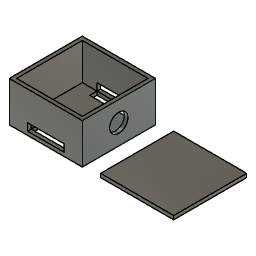
Caja Prototipo 1 v1 (Autodesk Fusion 360 design; units mm, degrees)
Autodesk Fusion 360 part; units mm, degrees
sketch "Boceto1" plane through (0, 0, 0) normal (0, 0, 1) x (1, 0, 0)
  line L0 (100, 100) -> (-100, 100)
  line L1 (-100, 100) -> (-100, -100)
  line L2 (-100, -100) -> (100, -100)
  line L3 (100, -100) -> (100, 100)
  line L4 (100, 100) -> (-100, -100) construction
  line L5 (-100, 100) -> (100, -100) construction
  dimension "L_base" = 200
  constraint horizontal L0
  constraint perpendicular L0 L1
  constraint parallel L0 L2
  constraint parallel L1 L3
  constraint coincident L4 origin
  constraint coincident L5 origin
  constraint equal L0 L1
  measures "L_base" distance of L0.end L1.end
extrude "Extruir1" add sketch "Boceto1" along normal blind 10 makes body 1
sketch "Boceto2" plane through (0, 0, 10) normal (0, 0, 1) x (-1, 0, 0)
  line L0 (-100, 100) -> (-100, -100)
  line L1 (-100, -100) -> (100, -100)
  line L2 (100, -100) -> (100, 100)
  line L3 (100, 100) -> (-100, 100)
  line L4 (100, -100) -> (90, -100)
  line L5 (90, -100) -> (90, 100)
  line L6 (90, 100) -> (100, 100)
  line L7 (100, 100) -> (100, -100)
  line L8 (90, -90) -> (-100, -90)
  line L9 (-100, -90) -> (-100, -100)
  line L10 (-100, -100) -> (90, -100)
  line L11 (90, -100) -> (90, -90)
  line L12 (-90, -90) -> (-100, -90)
  line L13 (-100, -90) -> (-100, 100)
  line L14 (-100, 100) -> (-90, 100)
  line L15 (-90, 100) -> (-90, -90)
  line L16 (-90, 100) -> (90, 100)
  line L17 (90, 100) -> (90, 90)
  line L18 (90, 90) -> (-90, 90)
  line L19 (-90, 90) -> (-90, 100)
  dimension "d4" = 10
  dimension "d5" = 10
  dimension "d6" = 10
  dimension "d7" = 10
  constraint horizontal L4
  constraint vertical L5
  constraint horizontal L6
  constraint vertical L7
  constraint coincident L3 L5.end
  constraint coincident L1.end L2.start
  constraint horizontal L8
  constraint vertical L9
  constraint horizontal L10
  constraint vertical L11
  constraint coincident L0.end L1.start
  constraint coincident L5 L8.start
  constraint horizontal L12
  constraint vertical L13
  constraint horizontal L14
  constraint vertical L15
  constraint coincident L0.start L3.end
  constraint coincident L8 L12.start
  constraint horizontal L16
  constraint vertical L17
  constraint horizontal L18
  constraint vertical L19
  constraint coincident L5 L17.end
  measures "d4" distance of L5 L7
  measures "d5" distance of L8 L10
  measures "d6" distance of L13 L15
  measures "d7" distance of L16 L18
extrude "Extruir2" add sketch "Boceto2" along normal blind 100 contours L0 L3 L8 L12 L13 L14 L15 L19 | L0 L1 L5 L8 L9 L10 L11 L12 | L3 L5 L15 L16 L17 L18 L19 | L1 L2 L3 L4 L5 L6 L7 L11 L17 bodies 1
sketch "Boceto4" plane through (100, 0, 0) normal (1, 0, 0) x (0, 1, 0)
  line L0 (-100, 0) -> (100, 0)
  line L1 (100, 0) -> (100, 110)
  line L2 (100, 110) -> (-100, 110)
  line L3 (-100, 110) -> (-100, 0)
hole "Agujero1" at (100, -0.0759, 55.0508) direction (-1, 0, 0) diameter 50 depth 10 tip angle 118 bodies 1
sketch "Boceto5" plane through (0, 0, 0) normal (0, 0, 1) x (1, 0, 0)
  line L0 (150, 100) -> (350, 100)
  line L1 (350, 100) -> (350, -100)
  line L2 (350, -100) -> (150, -100)
  line L3 (150, -100) -> (150, 100)
  line L4 (150, 100) -> (350, -100) construction
  line L5 (350, 100) -> (150, -100) construction
  line L6 (100, 100) -> (-100, 100)
  point P0 (250, 0)
  dimension "d13" = 250
  dimension "d14" = 200
  constraint horizontal L0
  constraint perpendicular L0 L1
  constraint parallel L0 L2
  constraint parallel L1 L3
  constraint coincident L4 P0
  constraint coincident L5 P0
  constraint equal L1 L6
  constraint equal L0 L6
  constraint horizontal origin P0
  measures "d13" distance of origin P0
  measures "d14" distance of L0.end L1.end
extrude "Extruir3" add sketch "Boceto5" along normal blind 10 separate body makes body 2
sketch "Boceto6" plane through (0, -100, 0) normal (0, -1, 0) x (1, 0, 0)
  line L0 (-100, 0) -> (100, 0)
  line L1 (100, 0) -> (100, 110)
  line L2 (100, 110) -> (-100, 110)
  line L3 (-100, 110) -> (-100, 0)
  line L4 (0, 0) -> (0, 10)
  line L5 (50, 10) -> (-50, 10)
  line L6 (-50, 10) -> (-50, 30)
  line L7 (-50, 30) -> (50, 30)
  line L8 (50, 30) -> (50, 10)
  line L9 (50, 10) -> (-50, 30) construction
  line L10 (-50, 10) -> (50, 30) construction
  point P0 (0, 20)
  dimension "d17" = 10
  dimension "d18" = 20
  dimension "d19" = 100
  constraint coincident L4.start origin
  constraint perpendicular L0 L4
  constraint horizontal L5
  constraint perpendicular L5 L6
  constraint parallel L5 L7
  constraint parallel L6 L8
  constraint coincident L9 P0
  constraint coincident L10 P0
  constraint midpoint L10 P0
  constraint coincident L4.end L5
  constraint vertical L4.start P0
  measures "d17" distance of L4.start L4.end
  measures "d18" distance of L5.end L6.end
  measures "d19" distance of L6.end L7.end
extrude "Extruir4" cut sketch "Boceto6" along normal through all and the other way through all contours L5 L6 L7 L8 bodies 1
sketch "Boceto7" plane through (0, 0, 10) normal (0, 0, 1) x (-1, 0, 0)
  line L0 (50, -90) -> (90, -90)
  line L1 (90, -90) -> (90, 90)
  line L2 (90, 90) -> (50, 90)
  line L3 (50, 90) -> (50, 100)
  line L4 (50, 100) -> (-50, 100)
  line L5 (-50, 100) -> (-50, 90)
  line L6 (-50, 90) -> (-90, 90)
  line L7 (-90, 90) -> (-90, -90)
  line L8 (-90, -90) -> (-50, -90)
  line L9 (-50, -90) -> (-50, -100)
  line L10 (-50, -100) -> (50, -100)
  line L11 (50, -100) -> (50, -90)
  line L12 (50, -90) -> (-50, -90)
  line L13 (-50, -90) -> (-50, -70)
  line L14 (-50, -70) -> (50, -70)
  line L15 (50, -70) -> (50, -90)
  line L16 (50, 90) -> (-50, 90)
  line L17 (-50, 90) -> (-50, 70)
  line L18 (-50, 70) -> (50, 70)
  line L19 (50, 70) -> (50, 90)
  point P0 (50, -90)
  point P1 (-50, -90)
  point P2 (50, 90)
  point P3 (-50, 90)
  dimension "d21" = 100
  dimension "d22" = 20
  constraint coincident P0 L0.start
  constraint coincident P1 L8.end
  constraint coincident P2 L2.end
  constraint coincident P3 L5.end
  constraint horizontal L12
  constraint vertical L13
  constraint horizontal L14
  constraint vertical L15
  constraint horizontal L16
  constraint vertical L17
  constraint horizontal L18
  constraint vertical L19
  constraint equal L13 L17
  constraint equal L14 L18
  measures "d21" distance of L13.end L14.end
  measures "d22" distance of P1 L13.end
extrude "Extruir5" cut sketch "Boceto7" against normal up to surface (10 mm away) contours L12 L13 L14 L15 | L16 L17 L18 L19 bodies 1
